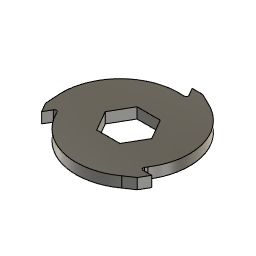
broyeuse V3 v5 (Autodesk Fusion 360 archive; units mm, degrees)
design "Dent A"
Autodesk Fusion 360 part; units mm, degrees
(part 1 of 5)
sketch "Sketch1" plane through (0, 0, 0) normal (0, 0, 1) x (1, 0, 0)
  circle A0 centre (0, 0) radius 25
  dimension "d4" = 50
  constraint coincident A0.centre origin
  measures "d4" diameter of A0
extrude "Extrude1" add sketch "Sketch1" along normal blind 5
sketch "Sketch2" plane through (0, 0, 5) normal (0, 0, 1) x (-1, 0, 0)
  circle A0 centre (0, 0) radius 25
  line L0 (5.4848, -9.5) -> (10.9697, 0)
  line L1 (10.9697, 0) -> (5.4848, 9.5)
  line L2 (5.4848, 9.5) -> (-5.4848, 9.5)
  line L3 (-5.4848, 9.5) -> (-10.9697, 0)
  line L4 (-10.9697, 0) -> (-5.4848, -9.5)
  line L5 (-5.4848, -9.5) -> (5.4848, -9.5)
  dimension "d7" = 19
  constraint coincident A0.centre origin
  measures "d7" distance of L0 L3
extrude "Extrude2" cut sketch "Sketch2" against normal through all contours L0 L1 L2 L3 L4 L5
sketch "Sketch3" plane through (0, 0, 5) normal (0, 0, 1) x (-1, 0, 0)
  line L0 (-10.9697, 0) -> (-5.4848, 9.5)
  line L1 (-5.4848, 9.5) -> (5.4848, 9.5)
  line L2 (5.4848, 9.5) -> (10.9697, 0)
  line L3 (10.9697, 0) -> (5.4848, -9.5)
  line L4 (5.4848, -9.5) -> (-5.4848, -9.5)
  line L5 (-5.4848, -9.5) -> (-10.9697, 0)
  circle A0 centre (0, 0) radius 25
  line L6 (0, -9.5) -> (0, -34) construction
  line L7 (0, -30) -> (-3.0461, -24.8137)
  line L8 (0, 0) -> (-21.6506, 12.5) construction
  arc A1 (-21.6506, 12.5) -> (0, -30) centre (1.3758, -2.5344) ccw
  line L9 (0, -30) -> (-5, -30)
  line L10 (-5, -30) -> (-11.5934, -26.7842)
  dimension "d9" = 120
  dimension "d10" = 55
  dimension "d11" = 30
  dimension "d14" = 5
  dimension "d16" = 154
  constraint midpoint L4 L6.start
  constraint perpendicular L4 L6
  constraint coincident L6 L7.start
  constraint coincident A0 L7.end
  constraint coincident A0.centre L8.start
  constraint coincident A0 L8.end
  constraint perpendicular L6 L9
  constraint coincident A1 L10.end
  measures "d9" angle of L6 L8
  measures "d10" diameter of A1
  measures "d11" distance of L7.start A0.centre
  measures "d14" distance of L7.start L9.end
  measures "d16" angle of L9 L10
extrude "Extrude3" add sketch "Sketch3" against normal blind 5 contours A0 L7 A1 L10 | A1 L10 | A1 L9 L10
pattern_circular "C-Pattern1" count 3 over 360 about axis through (0, 0, 1.75) along (0, 0, 1) of "Extrude3"
fillet "Fillet1" radius 1 3 edges at (19.9663, -15.0449, 2.5) (3.0461, 24.8137, 2.5) (-23.0124, -9.7689, 2.5)
sketch "Sketch4" plane through (0, 0, 5) normal (0, 0, 1) x (-1, 0, 0)
  line L0 (-10.9697, 0) -> (-5.4848, 9.5)
  line L1 (-5.4848, 9.5) -> (5.4848, 9.5)
  line L2 (5.4848, 9.5) -> (10.9697, 0)
  line L3 (10.9697, 0) -> (5.4848, -9.5)
  line L4 (5.4848, -9.5) -> (-5.4848, -9.5)
  line L5 (-5.4848, -9.5) -> (-10.9697, 0)
  arc A0 (-1.1597, -24.9731) -> (0, -25) centre (0, 0) ccw
  arc A1 (0, -25) -> (28.8493, 5.3994) centre (1.507, 2.4587) ccw
  line L6 (28.8493, 5.3994) -> (28.4808, 10.6699)
  line L7 (28.4808, 10.6699) -> (25.9808, 15)
  line L8 (25.9808, 15) -> (23.9652, 11.448)
  arc A2 (22.2072, 11.4822) -> (23.9652, 11.448) centre (23.0955, 11.9415) ccw
  arc A3 (22.2072, 11.4822) -> (21.6506, 12.5) centre (0, 0) ccw
  arc A4 (21.6506, 12.5) -> (-19.1007, 22.2845) centre (-2.8828, 0.0758) ccw
  line L9 (-19.1007, 22.2845) -> (-23.4808, 19.3301)
  line L10 (-23.4808, 19.3301) -> (-25.9808, 15)
  line L11 (-25.9808, 15) -> (-21.8968, 15.0305)
  arc A5 (-21.0475, 13.4909) -> (-21.8968, 15.0305) centre (-21.8894, 14.0305) ccw
  arc A6 (-21.0475, 13.4909) -> (-21.6506, 12.5) centre (0, 0) ccw
  arc A7 (-21.6506, 12.5) -> (-9.7486, -27.6839) centre (1.3758, -2.5344) ccw
  line L12 (-9.7486, -27.6839) -> (-5, -30)
  line L13 (-5, -30) -> (0, -30)
  line L14 (0, -30) -> (-2.0683, -26.4785)
  arc A8 (-1.1597, -24.9731) -> (-2.0683, -26.4785) centre (-1.2061, -25.972) ccw
  line L15 (0, 38) -> (0, -40)
  constraint vertical L15
equation "hexa_dent = 19 mm"
equation "hexa_axe = 19 mm"
equation "d7 = hexa_dent"

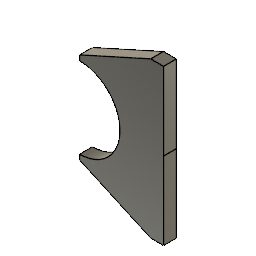
design "entretoise B"
Autodesk Fusion 360 part; units mm, degrees
sketch "Sketch1" plane through (0, 0, 0) normal (0, 1, 0) x (1, 0, 0)
  circle A0 centre (0, 0) radius 14.5 construction
  line L0 (0, -15.6) -> (0, -17.6)
  arc A1 (0, -15.6) -> (15.6, 0) centre (0, 0) ccw
  line L1 (0, -17.6) -> (27.5, -30)
  line L2 (0, 0) -> (15.6, 0) construction
  line L3 (27.5, -30) -> (32.5, -30)
  line L4 (32.5, -30) -> (32.5, 0)
  line L5 (0, -15.6) -> (0, 0) construction
  line L6 (0, 15.6) -> (0, 17.6)
  arc A2 (15.6, 0) -> (0, 15.6) centre (0, 0) ccw
  line L7 (0, 17.6) -> (27.5, 30)
  line L8 (27.5, 30) -> (32.5, 30)
  line L9 (32.5, 30) -> (32.5, 0)
  dimension "d1" = 29
  dimension "d2" = 2
  dimension "d3" = 30
  dimension "d4" = 32.5
  dimension "d5" = 15.6
  dimension "d6" = 5
  constraint coincident A0.centre A1.centre
  constraint horizontal L2
  constraint horizontal L3
  constraint perpendicular L3 L4
  constraint vertical L0
  constraint parallel L0 L5
  constraint symmetric L0.end L2 L6.end
  constraint symmetric L0.start L2 L6.start
  constraint symmetric A1 L2 A2
  constraint symmetric L1.end L2 L7.end
  constraint symmetric L2 A1.end A2.start
  constraint symmetric L2 L3.end L8.end
  constraint symmetric L2 L4.end L9.end
  measures "d1" diameter of A0
  measures "d2" distance of L0.end L0.start
  measures "d3" distance of L2 L3
  measures "d4" distance of A0.centre L4
  measures "d5" radius of A1
  measures "d6" distance of L1.end L3.end
extrude "Extrude1" add sketch "Sketch1" along normal blind 5

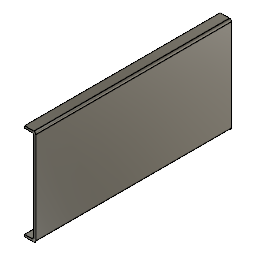
design "Flan"
Autodesk Fusion 360 part; units mm, degrees
sketch "Sketch1" plane through (0, 0, 0) normal (0, 1, 0) x (1, 0, 0)
  line L0 (-8.6431, -45) -> (0.9933, -45)
  line L1 (0.9933, -45) -> (0.9933, 49)
  line L2 (0.9933, 49) -> (-8.6431, 49)
  line L3 (-8.6431, -47.1) -> (3.0933, -47.1)
  line L4 (3.0933, -47.1) -> (3.0933, 51.1)
  line L5 (3.0933, 51.1) -> (-8.6431, 51.1)
  line L6 (-8.6431, -45) -> (-8.6431, -47.1)
  line L7 (-8.6431, 51.1) -> (-8.6431, 49)
  dimension "d1" = 94
  dimension "d2" = 2.1
  constraint horizontal L0
  constraint perpendicular L1 L2
  constraint vertical L1
  constraint equal L0 L2
  constraint perpendicular L2 L7
  measures "d1" distance of L0.end L1.end
extrude "Extrude1" add sketch "Sketch1" along normal blind 200
fillet "Fillet1" radius 2 1 edges at (3.0933, 100, 47.1)
fillet "Fillet1" radius 2 3 edges at (3.0933, 100, -51.1) (0.9933, 100, -49) (0.9933, 100, 45)

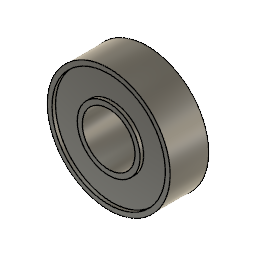
design "Q6202"
Autodesk Fusion 360 part; units mm, degrees
sketch "Sketch1" plane through (0, 0, 0) normal (0, 1, 0) x (1, 0, 0)
  circle A0 centre (0, 0) radius 17.5
  circle A1 centre (0, 0) radius 7.5
  dimension "d1" = 15
  dimension "d2" = 35
  constraint coincident A0.centre A1.centre
  constraint concentric A0 A1
  measures "d1" diameter of A1
  measures "d2" diameter of A0
extrude "Extrude1" add sketch "Sketch1" along normal blind 11
sketch "Sketch2" plane through (0, 0, 0) normal (0, -1, 0) x (1, 0, 0)
  circle A0 centre (0, 0) radius 7.5
  circle A1 centre (0, 0) radius 17.5
  circle A2 centre (0, 0) radius 8.9443
  circle A3 centre (0, 0) radius 16.1245
  constraint concentric A0 A2
  constraint concentric A2 A3
extrude "Extrude2" cut sketch "Sketch2" against normal blind 1 contours A3
ref_plane "WorkPlane1" through (0, 5.5, 0) normal (0, -1, 0) x (-1, 0, 0)
mirror "Mirror1" about plane through (0, 5.5, 0) normal (0, -1, 0) of "Extrude2"

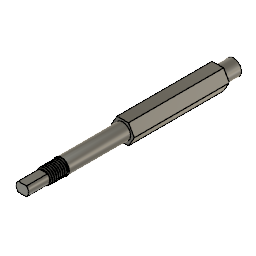
design "axe B"
Autodesk Fusion 360 part; units mm, degrees
sketch "Sketch1" plane through (0, 0, 0) normal (0, 1, 0) x (1, 0, 0)
  line L0 (5.4848, -9.5) -> (10.9697, 0)
  line L1 (10.9697, 0) -> (5.4848, 9.5)
  line L2 (5.4848, 9.5) -> (-5.4848, 9.5)
  line L3 (-5.4848, 9.5) -> (-10.9697, 0)
  line L4 (-10.9697, 0) -> (-5.4848, -9.5)
  line L5 (-5.4848, -9.5) -> (5.4848, -9.5)
  dimension "d1" = 19
  measures "d1" distance of L1 L4
extrude "Extrude1" add sketch "Sketch1" along normal blind 90
sketch "Sketch2" plane through (0, 0, 0) normal (0, -1, 0) x (1, 0, 0)
  line L0 (5.4848, 9.5) -> (-5.4848, 9.5)
  line L1 (-5.4848, 9.5) -> (-10.9697, 0)
  line L2 (-10.9697, 0) -> (-5.4848, -9.5)
  line L3 (-5.4848, -9.5) -> (5.4848, -9.5)
  line L4 (5.4848, -9.5) -> (10.9697, 0)
  line L5 (10.9697, 0) -> (5.4848, 9.5)
  circle A0 centre (0, 0) radius 7.5
  dimension "d4" = 15
  constraint coincident A0.centre origin
  measures "d4" diameter of A0
extrude "Extrude2" add sketch "Sketch2" along normal blind 58 contours A0
sketch "Sketch3" plane through (0, -58, 0) normal (0, -1, 0) x (1, 0, 0)
  circle A0 centre (0, 0) radius 7.5
  circle A1 centre (0, 0) radius 7
  dimension "d7" = 14
  constraint concentric A0 A1
  measures "d7" diameter of A1
extrude "Extrude3" add sketch "Sketch3" along normal blind 17 contours A1
thread "Thread1" "ISO Metric profile 14.0 M14x2 6g" major diameter 13.822 minor diameter 11.534 pitch 2 angle 60 modelled right hand crest width 0.2847 on face at (6.9913, -69.3333, -0.3489) crest through (6.911, -57.5, 0)
sketch "Sketch4" plane through (0, 90, 0) normal (0, 1, 0) x (-1, 0, 0)
  line L0 (5.4848, 9.5) -> (-5.4848, 9.5)
  line L1 (-5.4848, 9.5) -> (-10.9697, 0)
  line L2 (-10.9697, 0) -> (-5.4848, -9.5)
  line L3 (-5.4848, -9.5) -> (5.4848, -9.5)
  line L4 (5.4848, -9.5) -> (10.9697, 0)
  line L5 (10.9697, 0) -> (5.4848, 9.5)
  circle A0 centre (0, 0) radius 7.5
  dimension "d10" = 15
  constraint coincident A0.centre origin
  measures "d10" diameter of A0
extrude "Extrude4" add sketch "Sketch4" along normal blind 15 contours A0
sketch "Sketch5" plane through (0, -75, 0) normal (0, -1, 0) x (1, 0, 0)
  spline S0 degree 3 poles (-3.3483, 4.6955) (-4.0071, 4.3146) (-4.5838, 3.8067) (-5.5311, 2.5793) (-5.8844, 1.8654) (-6.3098, 0.3166) (-6.3676, -0.506) (-6.1666, -2.1557) (-5.8992, -2.9654) (-5.1959, -4.2209) (-4.8371, -4.6975) (-3.9949, -5.5534) (-3.5129, -5.9264) (-2.9883, -6.2315) knots 0 0 0 0 0.228303 0.228303 0.464774 0.464774 0.709409 0.709409 0.962206 0.962206 1.139841 1.139841 1.321288 1.321288 1.321288 1.321288
  arc A0 (-2.9883, -6.2315) -> (2.9883, -6.2315) centre (0, 0) ccw
  spline S1 degree 3 poles (2.9883, -6.2315) (3.7522, -5.7873) (4.4234, -5.2003) (5.482, -3.8207) (5.8675, -3.048) (6.3085, -1.4236) (6.3697, -0.5904) (6.1676, 1.0246) (5.9167, 1.7919) (5.2631, 2.9496) (4.9429, 3.3747) (4.2065, 4.1187) (3.7959, 4.4367) (3.3483, 4.6955) knots 0 0 0 0 0.265106 0.265106 0.522028 0.522028 0.770763 0.770763 1.011307 1.011307 1.170725 1.170725 1.326339 1.326339 1.326339 1.326339
  arc A1 (3.3483, 4.6955) -> (-3.3483, 4.6955) centre (0, 0) ccw
  circle A2 centre (0, 0) radius 6
  dimension "d13" = 12
  constraint coincident A0.centre A1.centre
  measures "d13" diameter of A2
extrude "Extrude5" add sketch "Sketch5" along normal blind 20 contours S0 S1 A1 A2 | S0 S1 A1 A2
sketch "Sketch6" plane through (0, -95, 0) normal (0, -1, 0) x (1, 0, 0)
  circle A0 centre (0, 0) radius 6
  line L0 (0, 0) -> (0, 6) construction
  line L1 (-8, 9.5) -> (10.7231, 9.5)
  line L2 (10.7231, 9.5) -> (10.7231, 4.5)
  line L3 (10.7231, 4.5) -> (-8, 4.5)
  line L4 (-8, 4.5) -> (-8, 9.5)
  line L5 (0, 0) -> (17.434, 0) construction
  line L6 (10.7231, -4.5) -> (-8, -4.5)
  line L7 (-8, -4.5) -> (-8, -9.5)
  line L8 (-8, -9.5) -> (10.7231, -9.5)
  line L9 (10.7231, -9.5) -> (10.7231, -4.5)
  dimension "d16" = 5
  dimension "d17" = 1.5
  constraint coincident A0.centre L0.start
  constraint vertical L0
  constraint horizontal L1
  constraint vertical L2
  constraint horizontal L3
  constraint vertical L4
  constraint coincident A0 L0.end
  constraint perpendicular L0 L5
  constraint symmetric L1.start L5 L7.end
  constraint symmetric L1.end L5 L8.end
  constraint symmetric L2.end L5 L6.start
  constraint symmetric L3.end L5 L6.end
  measures "d16" distance of L1.end L2.end
  measures "d17" distance of L0.end L3
extrude "Extrude6" cut sketch "Sketch6" against normal blind 20 contours A0 L3 | A0 L6

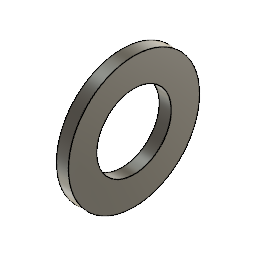
design "rondelle étroite M14 forme Z"
Autodesk Fusion 360 part; units mm, degrees
sketch "Sketch1" plane through (0, 0, 0) normal (1, 0, 0) x (0, 1, 0)
  circle A0 centre (0, 0) radius 7.65
  circle A1 centre (0, 0) radius 13.5
  dimension "d1" = 15.3
  dimension "d2" = 27
  constraint coincident A0.centre A1.centre
  measures "d1" diameter of A0
  measures "d2" diameter of A1
extrude "Extrude1" add sketch "Sketch1" along normal blind 2.5

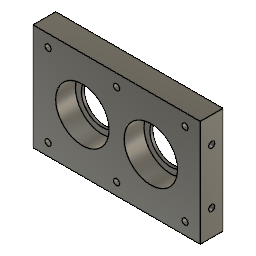
design "Plaque facade A"
Autodesk Fusion 360 part; units mm, degrees
sketch "Sketch1" plane through (0, 0, 0) normal (0, 1, 0) x (1, 0, 0)
  circle A0 centre (-22.5, 0) radius 13.6
  circle A1 centre (22.5, 0) radius 13.6
  line L0 (-22.5, 0) -> (22.5, 0) construction
  line L1 (0, 0) -> (0, -35) construction
  line L2 (-55, -35) -> (55, -35)
  line L3 (55, -35) -> (55, 35)
  line L4 (55, 35) -> (-55, 35)
  line L5 (-55, 35) -> (-55, -35)
  line L6 (-55, 0) -> (-22.5, 0) construction
  dimension "d1" = 27.2
  dimension "d2" = 45
  dimension "d3" = 70
  dimension "d4" = 110
  constraint equal A0 A1
  constraint coincident A0.centre L0.start
  constraint coincident A1.centre L0.end
  constraint horizontal L0
  constraint midpoint L0 L1.start
  constraint perpendicular L0 L1
  constraint coincident L1.start origin
  constraint horizontal L2
  constraint vertical L3
  constraint horizontal L4
  constraint vertical L5
  constraint midpoint L5 L6.start
  constraint perpendicular L5 L6
  constraint midpoint L1.end L2
  measures "d1" diameter of A0
  measures "d2" distance of A0.centre A1.centre
  measures "d3" distance of L2.start L4.end
  measures "d4" distance of L2.start L2.end
extrude "Extrude1" add sketch "Sketch1" along normal blind 15
sketch "Sketch2" plane through (0, 0, 0) normal (0, -1, 0) x (1, 0, 0)
  circle A0 centre (-22.5, 0) radius 13.6
  circle A1 centre (22.5, 0) radius 13.6
  line L0 (-55, 35) -> (-55, -35)
  line L1 (-55, -35) -> (55, -35)
  line L2 (55, -35) -> (55, 35)
  line L3 (55, 35) -> (-55, 35)
  circle A2 centre (-22.5, 0) radius 17.5
  circle A3 centre (22.5, 0) radius 17.5
  dimension "d7" = 35
  constraint concentric A0 A2
  constraint concentric A1 A3
  constraint equal A2 A3
  measures "d7" diameter of A2
extrude "Extrude2" cut sketch "Sketch2" against normal blind 13 contours A2 | A3
sketch "Sketch3" plane through (55, 0, 0) normal (1, 0, 0) x (0, 1, 0)
  line L0 (0, 35) -> (0, -35)
  line L1 (0, -35) -> (15, -35)
  line L2 (15, -35) -> (15, 35)
  line L3 (15, 35) -> (0, 35)
  line L4 (7.5, 35) -> (7.5, -35) construction
  circle A0 centre (7.5, 18) radius 2
  circle A1 centre (7.5, -18) radius 2
  line L5 (7.5, 0) -> (33, 0) construction
  dimension "d10" = 4
  dimension "d11" = 18
  dimension "d12" = 18
  constraint midpoint L3 L4.start
  constraint midpoint L1 L4.end
  constraint coincident L4 A0.centre
  constraint coincident L4 A1.centre
  constraint equal A0 A1
  constraint midpoint L4 L5.start
  constraint perpendicular L2 L5
  measures "d10" diameter of A0
  measures "d11" distance of A0.centre L5
  measures "d12" distance of A1.centre L5.start
extrude "Extrude3" cut sketch "Sketch3" against normal blind 20 contours A0 | A1
ref_plane "WorkPlane1" through (0, 7.5, 0) normal (1, 0, 0) x (0, 0, -1)
mirror "Mirror1" about plane through (0, 7.5, 0) normal (1, 0, 0) of "Extrude3"
sketch "Sketch4" plane through (0, 0, 0) normal (0, -1, 0) x (1, 0, 0)
  circle A0 centre (-22.5, 0) radius 17.5
  circle A1 centre (22.5, 0) radius 17.5
  line L0 (-55, 35) -> (-55, -35)
  line L1 (-55, -35) -> (55, -35)
  line L2 (55, -35) -> (55, 35)
  line L3 (55, 35) -> (-55, 35)
  line L4 (-55, 27) -> (55, 27) construction
  circle A2 centre (0, 27) radius 2
  circle A3 centre (-45, 27) radius 2
  circle A4 centre (45, 27) radius 2
  line L5 (55, 0) -> (-55, 0) construction
  circle A5 centre (45, -27) radius 2
  circle A6 centre (0, -27) radius 2
  circle A7 centre (-45, -27) radius 2
  dimension "d16" = 4
  dimension "d17" = 10
  dimension "d18" = 10
  dimension "d20" = 8
  constraint coincident L0 L4.start
  constraint coincident L2 L4.end
  constraint perpendicular L2 L4
  constraint midpoint L4 A2.centre
  constraint coincident L4 A3.centre
  constraint coincident L4 A4.centre
  constraint equal A2 A4
  constraint equal A2 A3
  constraint midpoint L2 L5.start
  constraint midpoint L0 L5.end
  constraint symmetric A2 L5 A6
  constraint symmetric A3 L5 A7
  constraint symmetric A4 L5 A5
  measures "d16" diameter of A3
  measures "d17" distance of L0 A3.centre
  measures "d18" distance of L2 A4.centre
  measures "d20" distance of L3 L4
extrude "Extrude4" cut sketch "Sketch4" against normal through all contours A2 | A3 | A4 | A5 | A6 | A7
equation "d12 = d11"

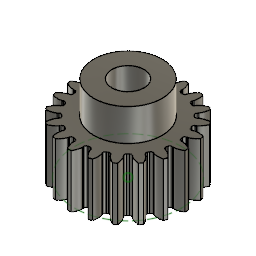
design "Engrenage 16D M2,5"
description: Spur Gear; Module: 2.5; Num Teeth: 20; Pressure Angle: 20.0; Backlash: 0.00 mm
Autodesk Fusion 360 part; units mm, degrees
sketch "Sketch1" plane through (0, 0, 0) normal (0, 0, 1) x (1, 0, 0) in component "Spur Gear (20 teeth)"
  circle A0 centre (0, 0) radius 21.9492
  circle A1 centre (0, 0) radius 7.5
extrude "Extrude1" add sketch "Sketch1" along normal blind 25 in component "Spur Gear (20 teeth)"
sketch "Sketch2" plane through (0, 0, 0) normal (0, 0, 1) x (1, 0, 0) in component "Spur Gear (20 teeth)"
  spline S0 degree 5 poles (23.3898, -2.192) (23.4016, -2.1931) (23.4251, -2.195) (23.4604, -2.1969) (23.5076, -2.1976) (23.5666, -2.1961) (23.6257, -2.1928) (23.6849, -2.1885) (23.7441, -2.1835) (23.8033, -2.1781) (23.8626, -2.1724) (23.9218, -2.166) (23.9811, -2.159) (24.0404, -2.151) (24.0996, -2.1423) (24.1589, -2.1327) (24.2182, -2.1224) (24.2775, -2.1116) (24.3368, -2.1003) (24.396, -2.0885) (24.4553, -2.0763) (24.5145, -2.0635) (24.5737, -2.0503) (24.6329, -2.0365) (24.6921, -2.0221) (24.7513, -2.0073) (24.8104, -1.992) (24.8696, -1.9762) (24.9287, -1.96) (24.9877, -1.9433) (25.0468, -1.9262) (25.1058, -1.9087) (25.1648, -1.8908) (25.2237, -1.8724) (25.2826, -1.8536) (25.3415, -1.8344) (25.4004, -1.8148) (25.4592, -1.7947) (25.518, -1.7743) (25.5767, -1.7535) (25.6354, -1.7323) (25.694, -1.7108) (25.7526, -1.6888) (25.8112, -1.6665) (25.8697, -1.6438) (25.9282, -1.6207) (25.9866, -1.5972) (26.045, -1.5734) (26.1034, -1.5493) (26.1616, -1.5248) (26.2199, -1.4999) (26.2781, -1.4747) (26.3362, -1.4491) (26.3943, -1.4232) (26.4523, -1.3969) (26.5102, -1.3704) (26.5682, -1.3434) (26.626, -1.3162) (26.6838, -1.2886) (26.7415, -1.2606) (26.7992, -1.2324) (26.8568, -1.2038) (26.9144, -1.1749) (26.9719, -1.1457) (27.0293, -1.1161) (27.0866, -1.0863) (27.1439, -1.0561) (27.2012, -1.0256) (27.2583, -0.9948) (27.3154, -0.9637) (27.3725, -0.9323) (27.418, -0.9069) (27.4522, -0.8877) (27.4749, -0.8749) (27.4863, -0.8685) knots 0 0 0 0 0 0 0.01428571 0.02857143 0.04285714 0.05714286 0.07142857 0.08571429 0.1 0.11428571 0.12857143 0.14285714 0.15714286 0.17142857 0.18571429 0.2 0.21428571 0.22857143 0.24285714 0.25714286 0.27142857 0.28571429 0.3 0.31428571 0.32857143 0.34285714 0.35714286 0.37142857 0.38571429 0.4 0.41428571 0.42857143 0.44285714 0.45714286 0.47142857 0.48571429 0.5 0.51428571 0.52857143 0.54285714 0.55714286 0.57142857 0.58571429 0.6 0.61428571 0.62857143 0.64285714 0.65714286 0.67142857 0.68571429 0.7 0.71428571 0.72857143 0.74285714 0.75714286 0.77142857 0.78571429 0.8 0.81428571 0.82857143 0.84285714 0.85714286 0.87142857 0.88571429 0.9 0.91428571 0.92857143 0.94285714 0.95714286 0.97142857 0.98571429 1 1 1 1 1 1
  spline S1 degree 5 poles (23.3898, 2.192) (23.4016, 2.1931) (23.4251, 2.195) (23.4604, 2.1969) (23.5076, 2.1976) (23.5666, 2.1961) (23.6257, 2.1928) (23.6849, 2.1885) (23.7441, 2.1835) (23.8033, 2.1781) (23.8626, 2.1724) (23.9218, 2.166) (23.9811, 2.159) (24.0404, 2.151) (24.0996, 2.1423) (24.1589, 2.1327) (24.2182, 2.1224) (24.2775, 2.1116) (24.3368, 2.1003) (24.396, 2.0885) (24.4553, 2.0763) (24.5145, 2.0635) (24.5737, 2.0503) (24.6329, 2.0365) (24.6921, 2.0221) (24.7513, 2.0073) (24.8104, 1.992) (24.8696, 1.9762) (24.9287, 1.96) (24.9877, 1.9433) (25.0468, 1.9262) (25.1058, 1.9087) (25.1648, 1.8908) (25.2237, 1.8724) (25.2826, 1.8536) (25.3415, 1.8344) (25.4004, 1.8148) (25.4592, 1.7947) (25.518, 1.7743) (25.5767, 1.7535) (25.6354, 1.7323) (25.694, 1.7108) (25.7526, 1.6888) (25.8112, 1.6665) (25.8697, 1.6438) (25.9282, 1.6207) (25.9866, 1.5972) (26.045, 1.5734) (26.1034, 1.5493) (26.1616, 1.5248) (26.2199, 1.4999) (26.2781, 1.4747) (26.3362, 1.4491) (26.3943, 1.4232) (26.4523, 1.3969) (26.5102, 1.3704) (26.5682, 1.3434) (26.626, 1.3162) (26.6838, 1.2886) (26.7415, 1.2606) (26.7992, 1.2324) (26.8568, 1.2038) (26.9144, 1.1749) (26.9719, 1.1457) (27.0293, 1.1161) (27.0866, 1.0863) (27.1439, 1.0561) (27.2012, 1.0256) (27.2583, 0.9948) (27.3154, 0.9637) (27.3725, 0.9323) (27.418, 0.9069) (27.4522, 0.8877) (27.4749, 0.8749) (27.4863, 0.8685) knots 0 0 0 0 0 0 0.01428571 0.02857143 0.04285714 0.05714286 0.07142857 0.08571429 0.1 0.11428571 0.12857143 0.14285714 0.15714286 0.17142857 0.18571429 0.2 0.21428571 0.22857143 0.24285714 0.25714286 0.27142857 0.28571429 0.3 0.31428571 0.32857143 0.34285714 0.35714286 0.37142857 0.38571429 0.4 0.41428571 0.42857143 0.44285714 0.45714286 0.47142857 0.48571429 0.5 0.51428571 0.52857143 0.54285714 0.55714286 0.57142857 0.58571429 0.6 0.61428571 0.62857143 0.64285714 0.65714286 0.67142857 0.68571429 0.7 0.71428571 0.72857143 0.74285714 0.75714286 0.77142857 0.78571429 0.8 0.81428571 0.82857143 0.84285714 0.85714286 0.87142857 0.88571429 0.9 0.91428571 0.92857143 0.94285714 0.95714286 0.97142857 0.98571429 1 1 1 1 1 1
  arc A0 (27.4863, -0.8685) -> (27.4863, 0.8685) centre (0, 0) ccw
  line L0 (21.8435, -2.048) -> (23.3898, -2.192)
  line L1 (21.8435, 2.048) -> (23.3898, 2.192)
  line L2 (21.8435, -2.048) -> (21.8435, 2.048)
  point P0 (23.6776, -2.1889)
  point P1 (23.9677, -2.1604)
  point P2 (24.2591, -2.1149)
  point P3 (24.5515, -2.0552)
  point P4 (24.8446, -1.9828)
  point P5 (25.1383, -1.8988)
  point P6 (25.4323, -1.8039)
  point P7 (25.7264, -1.6986)
  point P8 (26.0206, -1.5834)
  point P9 (26.3146, -1.4586)
  point P10 (26.6083, -1.3245)
  point P11 (26.9016, -1.1813)
  point P12 (27.1943, -1.0292)
  point P13 (23.6776, 2.1889)
  point P14 (23.9677, 2.1604)
  point P15 (24.2591, 2.1149)
  point P16 (24.5515, 2.0552)
  point P17 (24.8446, 1.9828)
  point P18 (25.1383, 1.8988)
  point P19 (25.4323, 1.8039)
  point P20 (25.7264, 1.6986)
  point P21 (26.0206, 1.5834)
  point P22 (26.3146, 1.4586)
  point P23 (26.6083, 1.3245)
  point P24 (26.9016, 1.1813)
  point P25 (27.1943, 1.0292)
extrude "Extrude2" add sketch "Sketch2" along normal blind 25 in component "Spur Gear (20 teeth)"
fillet "Fillet1" radius 1 2 edges at (21.8534, -2.049, 12.5) (21.8534, 2.049, 12.5) in component "Spur Gear (20 teeth)"
pattern_circular "C-Pattern1" count 20 over 360 about axis through (0, 0, 0) along (0, 0, 1) of "Extrude2", "Fillet1" in component "Spur Gear (20 teeth)"
sketch "Sketch3" plane through (0, 0, 0) normal (0, 0, 1) x (1, 0, 0) in component "Spur Gear (20 teeth)"
  circle A0 centre (0, 0) radius 25 construction
sketch "Sketch1 (2)" plane through (0, 0, 25) normal (0, 0, 1) x (-1, 0, 0)
  arc A0 (-21.6058, 3.8672) -> (-21.7434, 2.9987) centre (0, 0) ccw
  arc A1 (-22.8267, 2.1396) -> (-21.7434, 2.9987) centre (-22.734, 3.1353) ccw
  line L0 (-22.8267, 2.1396) -> (-23.3898, 2.192)
  spline S0 degree 5 poles (-23.3898, 2.192) (-23.4016, 2.1931) (-23.4251, 2.195) (-23.4604, 2.1969) (-23.5076, 2.1976) (-23.5666, 2.1961) (-23.6257, 2.1928) (-23.6849, 2.1885) (-23.7441, 2.1835) (-23.8033, 2.1781) (-23.8626, 2.1724) (-23.9218, 2.166) (-23.9811, 2.159) (-24.0404, 2.151) (-24.0996, 2.1423) (-24.1589, 2.1327) (-24.2182, 2.1224) (-24.2775, 2.1116) (-24.3368, 2.1003) (-24.396, 2.0885) (-24.4553, 2.0763) (-24.5145, 2.0635) (-24.5737, 2.0503) (-24.6329, 2.0365) (-24.6921, 2.0221) (-24.7513, 2.0073) (-24.8104, 1.992) (-24.8696, 1.9762) (-24.9287, 1.96) (-24.9877, 1.9433) (-25.0468, 1.9262) (-25.1058, 1.9087) (-25.1648, 1.8908) (-25.2237, 1.8724) (-25.2826, 1.8536) (-25.3415, 1.8344) (-25.4004, 1.8148) (-25.4592, 1.7947) (-25.518, 1.7743) (-25.5767, 1.7535) (-25.6354, 1.7323) (-25.694, 1.7108) (-25.7526, 1.6888) (-25.8112, 1.6665) (-25.8697, 1.6438) (-25.9282, 1.6207) (-25.9866, 1.5972) (-26.045, 1.5734) (-26.1034, 1.5493) (-26.1616, 1.5248) (-26.2199, 1.4999) (-26.2781, 1.4747) (-26.3362, 1.4491) (-26.3943, 1.4232) (-26.4523, 1.3969) (-26.5102, 1.3704) (-26.5682, 1.3434) (-26.626, 1.3162) (-26.6838, 1.2886) (-26.7415, 1.2606) (-26.7992, 1.2324) (-26.8568, 1.2038) (-26.9144, 1.1749) (-26.9719, 1.1457) (-27.0293, 1.1161) (-27.0866, 1.0863) (-27.1439, 1.0561) (-27.2012, 1.0256) (-27.2583, 0.9948) (-27.3154, 0.9637) (-27.3725, 0.9323) (-27.418, 0.9069) (-27.4522, 0.8877) (-27.4749, 0.8749) (-27.4863, 0.8685) knots 0 0 0 0 0 0 0.01428571 0.02857143 0.04285714 0.05714286 0.07142857 0.08571429 0.1 0.11428571 0.12857143 0.14285714 0.15714286 0.17142857 0.18571429 0.2 0.21428571 0.22857143 0.24285714 0.25714286 0.27142857 0.28571429 0.3 0.31428571 0.32857143 0.34285714 0.35714286 0.37142857 0.38571429 0.4 0.41428571 0.42857143 0.44285714 0.45714286 0.47142857 0.48571429 0.5 0.51428571 0.52857143 0.54285714 0.55714286 0.57142857 0.58571429 0.6 0.61428571 0.62857143 0.64285714 0.65714286 0.67142857 0.68571429 0.7 0.71428571 0.72857143 0.74285714 0.75714286 0.77142857 0.78571429 0.8 0.81428571 0.82857143 0.84285714 0.85714286 0.87142857 0.88571429 0.9 0.91428571 0.92857143 0.94285714 0.95714286 0.97142857 0.98571429 1 1 1 1 1 1
  arc A2 (-27.4863, 0.8685) -> (-27.4863, -0.8685) centre (0, 0) ccw
  spline S1 degree 5 poles (-27.4863, -0.8685) (-27.4749, -0.8749) (-27.4522, -0.8877) (-27.418, -0.9069) (-27.3725, -0.9323) (-27.3154, -0.9637) (-27.2583, -0.9948) (-27.2012, -1.0256) (-27.1439, -1.0561) (-27.0866, -1.0863) (-27.0293, -1.1161) (-26.9719, -1.1457) (-26.9144, -1.1749) (-26.8568, -1.2038) (-26.7992, -1.2324) (-26.7415, -1.2606) (-26.6838, -1.2886) (-26.626, -1.3162) (-26.5682, -1.3434) (-26.5102, -1.3704) (-26.4523, -1.3969) (-26.3943, -1.4232) (-26.3362, -1.4491) (-26.2781, -1.4747) (-26.2199, -1.4999) (-26.1616, -1.5248) (-26.1034, -1.5493) (-26.045, -1.5734) (-25.9866, -1.5972) (-25.9282, -1.6207) (-25.8697, -1.6438) (-25.8112, -1.6665) (-25.7526, -1.6888) (-25.694, -1.7108) (-25.6354, -1.7323) (-25.5767, -1.7535) (-25.518, -1.7743) (-25.4592, -1.7947) (-25.4004, -1.8148) (-25.3415, -1.8344) (-25.2826, -1.8536) (-25.2237, -1.8724) (-25.1648, -1.8908) (-25.1058, -1.9087) (-25.0468, -1.9262) (-24.9877, -1.9433) (-24.9287, -1.96) (-24.8696, -1.9762) (-24.8104, -1.992) (-24.7513, -2.0073) (-24.6921, -2.0221) (-24.6329, -2.0365) (-24.5737, -2.0503) (-24.5145, -2.0635) (-24.4553, -2.0763) (-24.396, -2.0885) (-24.3368, -2.1003) (-24.2775, -2.1116) (-24.2182, -2.1224) (-24.1589, -2.1327) (-24.0996, -2.1423) (-24.0404, -2.151) (-23.9811, -2.159) (-23.9218, -2.166) (-23.8626, -2.1724) (-23.8033, -2.1781) (-23.7441, -2.1835) (-23.6849, -2.1885) (-23.6257, -2.1928) (-23.5666, -2.1961) (-23.5076, -2.1976) (-23.4604, -2.1969) (-23.4251, -2.195) (-23.4016, -2.1931) (-23.3898, -2.192) knots -1 -1 -1 -1 -1 -1 -0.98571429 -0.97142857 -0.95714286 -0.94285714 -0.92857143 -0.91428571 -0.9 -0.88571429 -0.87142857 -0.85714286 -0.84285714 -0.82857143 -0.81428571 -0.8 -0.78571429 -0.77142857 -0.75714286 -0.74285714 -0.72857143 -0.71428571 -0.7 -0.68571429 -0.67142857 -0.65714286 -0.64285714 -0.62857143 -0.61428571 -0.6 -0.58571429 -0.57142857 -0.55714286 -0.54285714 -0.52857143 -0.51428571 -0.5 -0.48571429 -0.47142857 -0.45714286 -0.44285714 -0.42857143 -0.41428571 -0.4 -0.38571429 -0.37142857 -0.35714286 -0.34285714 -0.32857143 -0.31428571 -0.3 -0.28571429 -0.27142857 -0.25714286 -0.24285714 -0.22857143 -0.21428571 -0.2 -0.18571429 -0.17142857 -0.15714286 -0.14285714 -0.12857143 -0.11428571 -0.1 -0.08571429 -0.07142857 -0.05714286 -0.04285714 -0.02857143 -0.01428571 0 0 0 0 0 0
  line L1 (-23.3898, -2.192) -> (-22.8267, -2.1396)
  arc A3 (-21.7434, -2.9987) -> (-22.8267, -2.1396) centre (-22.734, -3.1353) ccw
  arc A4 (-21.7434, -2.9987) -> (-21.6058, -3.8672) centre (0, 0) ccw
  arc A5 (-22.3707, -5.019) -> (-21.6058, -3.8672) centre (-22.5902, -4.0434) ccw
  line L2 (-22.3707, -5.019) -> (-22.9224, -5.1431)
  spline S2 degree 5 poles (-22.9224, -5.1431) (-22.9339, -5.1457) (-22.9569, -5.1512) (-22.9911, -5.1603) (-23.0361, -5.1742) (-23.0918, -5.1939) (-23.147, -5.2153) (-23.2019, -5.2377) (-23.2567, -5.2607) (-23.3114, -5.2841) (-23.3659, -5.3079) (-23.4203, -5.3322) (-23.4745, -5.3573) (-23.5284, -5.3831) (-23.5821, -5.4098) (-23.6355, -5.4372) (-23.6888, -5.4653) (-23.7418, -5.4939) (-23.7947, -5.523) (-23.8474, -5.5525) (-23.9, -5.5824) (-23.9523, -5.6129) (-24.0046, -5.6438) (-24.0566, -5.6752) (-24.1085, -5.7071) (-24.1602, -5.7395) (-24.2117, -5.7724) (-24.263, -5.8056) (-24.3142, -5.8393) (-24.3653, -5.8734) (-24.4161, -5.9079) (-24.4668, -5.9428) (-24.5174, -5.9781) (-24.5678, -6.0138) (-24.618, -6.0499) (-24.6681, -6.0864) (-24.718, -6.1232) (-24.7677, -6.1604) (-24.8173, -6.198) (-24.8667, -6.2359) (-24.916, -6.2742) (-24.9651, -6.3129) (-25.0141, -6.3519) (-25.0629, -6.3912) (-25.1115, -6.4309) (-25.16, -6.4709) (-25.2083, -6.5112) (-25.2565, -6.5519) (-25.3045, -6.5929) (-25.3524, -6.6343) (-25.4001, -6.6759) (-25.4476, -6.7179) (-25.495, -6.7601) (-25.5422, -6.8027) (-25.5893, -6.8456) (-25.6362, -6.8888) (-25.683, -6.9323) (-25.7296, -6.9761) (-25.776, -7.0202) (-25.8223, -7.0646) (-25.8684, -7.1093) (-25.9144, -7.1543) (-25.9602, -7.1996) (-26.0058, -7.2452) (-26.0513, -7.291) (-26.0966, -7.3371) (-26.1418, -7.3835) (-26.1868, -7.4302) (-26.2316, -7.4772) (-26.2763, -7.5244) (-26.3208, -7.5719) (-26.3563, -7.6101) (-26.3829, -7.6389) (-26.4006, -7.6581) (-26.4094, -7.6678) knots 0 0 0 0 0 0 0.01428571 0.02857143 0.04285714 0.05714286 0.07142857 0.08571429 0.1 0.11428571 0.12857143 0.14285714 0.15714286 0.17142857 0.18571429 0.2 0.21428571 0.22857143 0.24285714 0.25714286 0.27142857 0.28571429 0.3 0.31428571 0.32857143 0.34285714 0.35714286 0.37142857 0.38571429 0.4 0.41428571 0.42857143 0.44285714 0.45714286 0.47142857 0.48571429 0.5 0.51428571 0.52857143 0.54285714 0.55714286 0.57142857 0.58571429 0.6 0.61428571 0.62857143 0.64285714 0.65714286 0.67142857 0.68571429 0.7 0.71428571 0.72857143 0.74285714 0.75714286 0.77142857 0.78571429 0.8 0.81428571 0.82857143 0.84285714 0.85714286 0.87142857 0.88571429 0.9 0.91428571 0.92857143 0.94285714 0.95714286 0.97142857 0.98571429 1 1 1 1 1 1
  arc A6 (-26.4094, -7.6678) -> (-25.8726, -9.3197) centre (0, 0) ccw
  spline S3 degree 5 poles (-25.8726, -9.3197) (-25.8598, -9.3223) (-25.8342, -9.3275) (-25.7958, -9.3352) (-25.7447, -9.3452) (-25.6807, -9.3575) (-25.6168, -9.3694) (-25.5529, -9.381) (-25.4891, -9.3924) (-25.4253, -9.4033) (-25.3615, -9.414) (-25.2977, -9.4244) (-25.234, -9.4344) (-25.1704, -9.4441) (-25.1067, -9.4535) (-25.0432, -9.4625) (-24.9796, -9.4712) (-24.9161, -9.4796) (-24.8527, -9.4877) (-24.7893, -9.4954) (-24.7259, -9.5028) (-24.6626, -9.5098) (-24.5994, -9.5165) (-24.5362, -9.5229) (-24.4731, -9.5289) (-24.41, -9.5345) (-24.347, -9.5398) (-24.2841, -9.5448) (-24.2212, -9.5494) (-24.1584, -9.5536) (-24.0956, -9.5575) (-24.033, -9.561) (-23.9704, -9.5642) (-23.9078, -9.5669) (-23.8454, -9.5693) (-23.783, -9.5713) (-23.7207, -9.573) (-23.6585, -9.5742) (-23.5964, -9.5751) (-23.5344, -9.5756) (-23.4724, -9.5756) (-23.4106, -9.5753) (-23.3488, -9.5746) (-23.2872, -9.5734) (-23.2257, -9.5718) (-23.1642, -9.5698) (-23.1029, -9.5674) (-23.0417, -9.5646) (-22.9806, -9.5613) (-22.9196, -9.5576) (-22.8587, -9.5535) (-22.798, -9.5488) (-22.7374, -9.5436) (-22.677, -9.5379) (-22.6167, -9.5318) (-22.5566, -9.5251) (-22.4966, -9.518) (-22.4367, -9.5104) (-22.377, -9.5024) (-22.3175, -9.4938) (-22.2581, -9.4846) (-22.199, -9.4746) (-22.1402, -9.4638) (-22.0817, -9.4523) (-22.0233, -9.44) (-21.9652, -9.4272) (-21.9072, -9.414) (-21.8494, -9.4004) (-21.7918, -9.3863) (-21.7346, -9.3711) (-21.6779, -9.3543) (-21.6333, -9.339) (-21.6003, -9.3263) (-21.5785, -9.3173) (-21.5677, -9.3126) knots -1 -1 -1 -1 -1 -1 -0.98571429 -0.97142857 -0.95714286 -0.94285714 -0.92857143 -0.91428571 -0.9 -0.88571429 -0.87142857 -0.85714286 -0.84285714 -0.82857143 -0.81428571 -0.8 -0.78571429 -0.77142857 -0.75714286 -0.74285714 -0.72857143 -0.71428571 -0.7 -0.68571429 -0.67142857 -0.65714286 -0.64285714 -0.62857143 -0.61428571 -0.6 -0.58571429 -0.57142857 -0.55714286 -0.54285714 -0.52857143 -0.51428571 -0.5 -0.48571429 -0.47142857 -0.45714286 -0.44285714 -0.42857143 -0.41428571 -0.4 -0.38571429 -0.37142857 -0.35714286 -0.34285714 -0.32857143 -0.31428571 -0.3 -0.28571429 -0.27142857 -0.25714286 -0.24285714 -0.22857143 -0.21428571 -0.2 -0.18571429 -0.17142857 -0.15714286 -0.14285714 -0.12857143 -0.11428571 -0.1 -0.08571429 -0.07142857 -0.05714286 -0.04285714 -0.02857143 -0.01428571 0 0 0 0 0 0
  line L3 (-21.5677, -9.3126) -> (-21.0483, -9.0887)
  arc A7 (-19.7526, -9.571) -> (-21.0483, -9.0887) centre (-20.6525, -10.007) ccw
  arc A8 (-19.7526, -9.571) -> (-19.3534, -10.3545) centre (0, 0) ccw
  arc A9 (-19.7248, -11.6862) -> (-19.3534, -10.3545) centre (-20.2351, -10.8262) ccw
  line L4 (-19.7248, -11.6862) -> (-20.2112, -11.9748)
  spline S4 degree 5 poles (-20.2112, -11.9748) (-20.2214, -11.9808) (-20.2415, -11.9931) (-20.2712, -12.0124) (-20.3098, -12.0395) (-20.3566, -12.0754) (-20.4025, -12.1128) (-20.4478, -12.1511) (-20.4928, -12.1899) (-20.5376, -12.2291) (-20.5821, -12.2686) (-20.6263, -12.3085) (-20.6701, -12.3491) (-20.7134, -12.3903) (-20.7562, -12.4323) (-20.7985, -12.4749) (-20.8405, -12.518) (-20.8821, -12.5616) (-20.9234, -12.6056) (-20.9644, -12.65) (-21.0051, -12.6947) (-21.0456, -12.7398) (-21.0857, -12.7854) (-21.1255, -12.8313) (-21.1649, -12.8777) (-21.2041, -12.9245) (-21.2429, -12.9717) (-21.2815, -13.0192) (-21.3198, -13.0671) (-21.3577, -13.1152) (-21.3955, -13.1638) (-21.4329, -13.2126) (-21.4701, -13.2618) (-21.507, -13.3113) (-21.5436, -13.3612) (-21.5799, -13.4113) (-21.616, -13.4618) (-21.6518, -13.5126) (-21.6874, -13.5636) (-21.7227, -13.615) (-21.7577, -13.6666) (-21.7925, -13.7185) (-21.827, -13.7708) (-21.8612, -13.8233) (-21.8952, -13.876) (-21.929, -13.9291) (-21.9625, -13.9824) (-21.9957, -14.0359) (-22.0287, -14.0898) (-22.0615, -14.1439) (-22.0939, -14.1982) (-22.1262, -14.2528) (-22.1582, -14.3077) (-22.1899, -14.3628) (-22.2215, -14.4181) (-22.2527, -14.4737) (-22.2837, -14.5295) (-22.3145, -14.5856) (-22.345, -14.6419) (-22.3753, -14.6984) (-22.4054, -14.7552) (-22.4352, -14.8121) (-22.4648, -14.8694) (-22.4941, -14.9268) (-22.5232, -14.9844) (-22.5521, -15.0423) (-22.5807, -15.1004) (-22.6091, -15.1587) (-22.6372, -15.2172) (-22.6651, -15.276) (-22.6928, -15.3349) (-22.7147, -15.3822) (-22.7311, -15.4178) (-22.7419, -15.4415) (-22.7473, -15.4534) knots 0 0 0 0 0 0 0.01428571 0.02857143 0.04285714 0.05714286 0.07142857 0.08571429 0.1 0.11428571 0.12857143 0.14285714 0.15714286 0.17142857 0.18571429 0.2 0.21428571 0.22857143 0.24285714 0.25714286 0.27142857 0.28571429 0.3 0.31428571 0.32857143 0.34285714 0.35714286 0.37142857 0.38571429 0.4 0.41428571 0.42857143 0.44285714 0.45714286 0.47142857 0.48571429 0.5 0.51428571 0.52857143 0.54285714 0.55714286 0.57142857 0.58571429 0.6 0.61428571 0.62857143 0.64285714 0.65714286 0.67142857 0.68571429 0.7 0.71428571 0.72857143 0.74285714 0.75714286 0.77142857 0.78571429 0.8 0.81428571 0.82857143 0.84285714 0.85714286 0.87142857 0.88571429 0.9 0.91428571 0.92857143 0.94285714 0.95714286 0.97142857 0.98571429 1 1 1 1 1 1
  arc A10 (-22.7473, -15.4534) -> (-21.7264, -16.8586) centre (0, 0) ccw
  spline S5 degree 5 poles (-21.7264, -16.8586) (-21.7134, -16.8572) (-21.6875, -16.8542) (-21.6486, -16.8496) (-21.5968, -16.8434) (-21.5322, -16.8353) (-21.4677, -16.8269) (-21.4034, -16.8182) (-21.3392, -16.8092) (-21.2751, -16.7999) (-21.2111, -16.7904) (-21.1473, -16.7805) (-21.0836, -16.7704) (-21.02, -16.7599) (-20.9566, -16.7492) (-20.8934, -16.7382) (-20.8302, -16.7268) (-20.7673, -16.7152) (-20.7044, -16.7032) (-20.6418, -16.691) (-20.5792, -16.6784) (-20.5169, -16.6656) (-20.4547, -16.6524) (-20.3926, -16.6389) (-20.3307, -16.6251) (-20.269, -16.611) (-20.2074, -16.5966) (-20.146, -16.5818) (-20.0848, -16.5668) (-20.0238, -16.5514) (-19.9629, -16.5357) (-19.9022, -16.5197) (-19.8417, -16.5033) (-19.7814, -16.4866) (-19.7212, -16.4696) (-19.6613, -16.4522) (-19.6015, -16.4345) (-19.542, -16.4165) (-19.4826, -16.3981) (-19.4235, -16.3794) (-19.3646, -16.3604) (-19.3059, -16.3409) (-19.2474, -16.3211) (-19.1891, -16.301) (-19.1311, -16.2805) (-19.0732, -16.2596) (-19.0157, -16.2383) (-18.9583, -16.2167) (-18.9012, -16.1948) (-18.8444, -16.1724) (-18.7878, -16.1496) (-18.7315, -16.1264) (-18.6754, -16.1028) (-18.6197, -16.0787) (-18.5643, -16.0542) (-18.5092, -16.0293) (-18.4543, -16.004) (-18.3997, -15.9783) (-18.3454, -15.9522) (-18.2914, -15.9256) (-18.2378, -15.8985) (-18.1847, -15.8708) (-18.1321, -15.8424) (-18.08, -15.8132) (-18.0283, -15.7835) (-17.977, -15.7534) (-17.9259, -15.7229) (-17.8751, -15.6921) (-17.8247, -15.6609) (-17.775, -15.6288) (-17.7263, -15.5953) (-17.6886, -15.567) (-17.6611, -15.5447) (-17.6432, -15.5294) (-17.6343, -15.5216) knots -1 -1 -1 -1 -1 -1 -0.98571429 -0.97142857 -0.95714286 -0.94285714 -0.92857143 -0.91428571 -0.9 -0.88571429 -0.87142857 -0.85714286 -0.84285714 -0.82857143 -0.81428571 -0.8 -0.78571429 -0.77142857 -0.75714286 -0.74285714 -0.72857143 -0.71428571 -0.7 -0.68571429 -0.67142857 -0.65714286 -0.64285714 -0.62857143 -0.61428571 -0.6 -0.58571429 -0.57142857 -0.55714286 -0.54285714 -0.52857143 -0.51428571 -0.5 -0.48571429 -0.47142857 -0.45714286 -0.44285714 -0.42857143 -0.41428571 -0.4 -0.38571429 -0.37142857 -0.35714286 -0.34285714 -0.32857143 -0.31428571 -0.3 -0.28571429 -0.27142857 -0.25714286 -0.24285714 -0.22857143 -0.21428571 -0.2 -0.18571429 -0.17142857 -0.15714286 -0.14285714 -0.12857143 -0.11428571 -0.1 -0.08571429 -0.07142857 -0.05714286 -0.04285714 -0.02857143 -0.01428571 0 0 0 0 0 0
  line L5 (-17.6343, -15.5216) -> (-17.2096, -15.1482)
  arc A11 (-15.8282, -15.2064) -> (-17.2096, -15.1482) centre (-16.5493, -15.8992) ccw
  arc A12 (-15.8282, -15.2064) -> (-15.2064, -15.8282) centre (0, 0) ccw
  arc A13 (-15.1482, -17.2096) -> (-15.2064, -15.8282) centre (-15.8992, -16.5493) ccw
  line L6 (-15.1482, -17.2096) -> (-15.5216, -17.6343)
  spline S6 degree 5 poles (-15.5216, -17.6343) (-15.5294, -17.6432) (-15.5447, -17.6611) (-15.567, -17.6886) (-15.5953, -17.7263) (-15.6288, -17.775) (-15.6609, -17.8247) (-15.6921, -17.8751) (-15.7229, -17.9259) (-15.7534, -17.977) (-15.7835, -18.0283) (-15.8132, -18.08) (-15.8424, -18.1321) (-15.8708, -18.1847) (-15.8985, -18.2378) (-15.9256, -18.2914) (-15.9522, -18.3454) (-15.9783, -18.3997) (-16.004, -18.4543) (-16.0293, -18.5092) (-16.0542, -18.5643) (-16.0787, -18.6197) (-16.1028, -18.6754) (-16.1264, -18.7315) (-16.1496, -18.7878) (-16.1724, -18.8444) (-16.1948, -18.9012) (-16.2167, -18.9583) (-16.2383, -19.0157) (-16.2596, -19.0732) (-16.2805, -19.1311) (-16.301, -19.1891) (-16.3211, -19.2474) (-16.3409, -19.3059) (-16.3604, -19.3646) (-16.3794, -19.4235) (-16.3981, -19.4826) (-16.4165, -19.542) (-16.4345, -19.6015) (-16.4522, -19.6613) (-16.4696, -19.7212) (-16.4866, -19.7814) (-16.5033, -19.8417) (-16.5197, -19.9022) (-16.5357, -19.9629) (-16.5514, -20.0238) (-16.5668, -20.0848) (-16.5818, -20.146) (-16.5966, -20.2074) (-16.611, -20.269) (-16.6251, -20.3307) (-16.6389, -20.3926) (-16.6524, -20.4547) (-16.6656, -20.5169) (-16.6784, -20.5792) (-16.691, -20.6418) (-16.7032, -20.7044) (-16.7152, -20.7673) (-16.7268, -20.8302) (-16.7382, -20.8934) (-16.7492, -20.9566) (-16.7599, -21.02) (-16.7704, -21.0836) (-16.7805, -21.1473) (-16.7904, -21.2111) (-16.7999, -21.2751) (-16.8092, -21.3392) (-16.8182, -21.4034) (-16.8269, -21.4677) (-16.8353, -21.5322) (-16.8434, -21.5968) (-16.8496, -21.6486) (-16.8542, -21.6875) (-16.8572, -21.7134) (-16.8586, -21.7264) knots 0 0 0 0 0 0 0.01428571 0.02857143 0.04285714 0.05714286 0.07142857 0.08571429 0.1 0.11428571 0.12857143 0.14285714 0.15714286 0.17142857 0.18571429 0.2 0.21428571 0.22857143 0.24285714 0.25714286 0.27142857 0.28571429 0.3 0.31428571 0.32857143 0.34285714 0.35714286 0.37142857 0.38571429 0.4 0.41428571 0.42857143 0.44285714 0.45714286 0.47142857 0.48571429 0.5 0.51428571 0.52857143 0.54285714 0.55714286 0.57142857 0.58571429 0.6 0.61428571 0.62857143 0.64285714 0.65714286 0.67142857 0.68571429 0.7 0.71428571 0.72857143 0.74285714 0.75714286 0.77142857 0.78571429 0.8 0.81428571 0.82857143 0.84285714 0.85714286 0.87142857 0.88571429 0.9 0.91428571 0.92857143 0.94285714 0.95714286 0.97142857 0.98571429 1 1 1 1 1 1
  arc A14 (-16.8586, -21.7264) -> (-15.4534, -22.7473) centre (0, 0) ccw
  spline S7 degree 5 poles (-15.4534, -22.7473) (-15.4415, -22.7419) (-15.4178, -22.7311) (-15.3822, -22.7147) (-15.3349, -22.6928) (-15.276, -22.6651) (-15.2172, -22.6372) (-15.1587, -22.6091) (-15.1004, -22.5807) (-15.0423, -22.5521) (-14.9844, -22.5232) (-14.9268, -22.4941) (-14.8694, -22.4648) (-14.8121, -22.4352) (-14.7552, -22.4054) (-14.6984, -22.3753) (-14.6419, -22.345) (-14.5856, -22.3145) (-14.5295, -22.2837) (-14.4737, -22.2527) (-14.4181, -22.2215) (-14.3628, -22.1899) (-14.3077, -22.1582) (-14.2528, -22.1262) (-14.1982, -22.0939) (-14.1439, -22.0615) (-14.0898, -22.0287) (-14.0359, -21.9957) (-13.9824, -21.9625) (-13.9291, -21.929) (-13.876, -21.8952) (-13.8233, -21.8612) (-13.7708, -21.827) (-13.7185, -21.7925) (-13.6666, -21.7577) (-13.615, -21.7227) (-13.5636, -21.6874) (-13.5126, -21.6518) (-13.4618, -21.616) (-13.4113, -21.5799) (-13.3612, -21.5436) (-13.3113, -21.507) (-13.2618, -21.4701) (-13.2126, -21.4329) (-13.1638, -21.3955) (-13.1152, -21.3577) (-13.0671, -21.3198) (-13.0192, -21.2815) (-12.9717, -21.2429) (-12.9245, -21.2041) (-12.8777, -21.1649) (-12.8313, -21.1255) (-12.7854, -21.0857) (-12.7398, -21.0456) (-12.6947, -21.0051) (-12.65, -20.9644) (-12.6056, -20.9234) (-12.5616, -20.8821) (-12.518, -20.8405) (-12.4749, -20.7985) (-12.4323, -20.7562) (-12.3903, -20.7134) (-12.3491, -20.6701) (-12.3085, -20.6263) (-12.2686, -20.5821) (-12.2291, -20.5376) (-12.1899, -20.4928) (-12.1511, -20.4478) (-12.1128, -20.4025) (-12.0754, -20.3566) (-12.0395, -20.3098) (-12.0124, -20.2712) (-11.9931, -20.2415) (-11.9808, -20.2214) (-11.9748, -20.2112) knots -1 -1 -1 -1 -1 -1 -0.98571429 -0.97142857 -0.95714286 -0.94285714 -0.92857143 -0.91428571 -0.9 -0.88571429 -0.87142857 -0.85714286 -0.84285714 -0.82857143 -0.81428571 -0.8 -0.78571429 -0.77142857 -0.75714286 -0.74285714 -0.72857143 -0.71428571 -0.7 -0.68571429 -0.67142857 -0.65714286 -0.64285714 -0.62857143 -0.61428571 -0.6 -0.58571429 -0.57142857 -0.55714286 -0.54285714 -0.52857143 -0.51428571 -0.5 -0.48571429 -0.47142857 -0.45714286 -0.44285714 -0.42857143 -0.41428571 -0.4 -0.38571429 -0.37142857 -0.35714286 -0.34285714 -0.32857143 -0.31428571 -0.3 -0.28571429 -0.27142857 -0.25714286 -0.24285714 -0.22857143 -0.21428571 -0.2 -0.18571429 -0.17142857 -0.15714286 -0.14285714 -0.12857143 -0.11428571 -0.1 -0.08571429 -0.07142857 -0.05714286 -0.04285714 -0.02857143 -0.01428571 0 0 0 0 0 0
  line L7 (-11.9748, -20.2112) -> (-11.6862, -19.7248)
  arc A15 (-10.3545, -19.3534) -> (-11.6862, -19.7248) centre (-10.8262, -20.2351) ccw
  arc A16 (-10.3545, -19.3534) -> (-9.571, -19.7526) centre (0, 0) ccw
  arc A17 (-9.0887, -21.0483) -> (-9.571, -19.7526) centre (-10.007, -20.6525) ccw
  line L8 (-9.0887, -21.0483) -> (-9.3126, -21.5677)
  spline S8 degree 5 poles (-9.3126, -21.5677) (-9.3173, -21.5785) (-9.3263, -21.6003) (-9.339, -21.6333) (-9.3543, -21.6779) (-9.3711, -21.7346) (-9.3863, -21.7918) (-9.4004, -21.8494) (-9.414, -21.9072) (-9.4272, -21.9652) (-9.44, -22.0233) (-9.4523, -22.0817) (-9.4638, -22.1402) (-9.4746, -22.199) (-9.4846, -22.2581) (-9.4938, -22.3175) (-9.5024, -22.377) (-9.5104, -22.4367) (-9.518, -22.4966) (-9.5251, -22.5566) (-9.5318, -22.6167) (-9.5379, -22.677) (-9.5436, -22.7374) (-9.5488, -22.798) (-9.5535, -22.8587) (-9.5576, -22.9196) (-9.5613, -22.9806) (-9.5646, -23.0417) (-9.5674, -23.1029) (-9.5698, -23.1642) (-9.5718, -23.2257) (-9.5734, -23.2872) (-9.5746, -23.3488) (-9.5753, -23.4106) (-9.5756, -23.4724) (-9.5756, -23.5344) (-9.5751, -23.5964) (-9.5742, -23.6585) (-9.573, -23.7207) (-9.5713, -23.783) (-9.5693, -23.8454) (-9.5669, -23.9078) (-9.5642, -23.9704) (-9.561, -24.033) (-9.5575, -24.0956) (-9.5536, -24.1584) (-9.5494, -24.2212) (-9.5448, -24.2841) (-9.5398, -24.347) (-9.5345, -24.41) (-9.5289, -24.4731) (-9.5229, -24.5362) (-9.5165, -24.5994) (-9.5098, -24.6626) (-9.5028, -24.7259) (-9.4954, -24.7893) (-9.4877, -24.8527) (-9.4796, -24.9161) (-9.4712, -24.9796) (-9.4625, -25.0432) (-9.4535, -25.1067) (-9.4441, -25.1704) (-9.4344, -25.234) (-9.4244, -25.2977) (-9.414, -25.3615) (-9.4033, -25.4253) (-9.3924, -25.4891) (-9.381, -25.5529) (-9.3694, -25.6168) (-9.3575, -25.6807) (-9.3452, -25.7447) (-9.3352, -25.7958) (-9.3275, -25.8342) (-9.3223, -25.8598) (-9.3197, -25.8726) knots 0 0 0 0 0 0 0.01428571 0.02857143 0.04285714 0.05714286 0.07142857 0.08571429 0.1 0.11428571 0.12857143 0.14285714 0.15714286 0.17142857 0.18571429 0.2 0.21428571 0.22857143 0.24285714 0.25714286 0.27142857 0.28571429 0.3 0.31428571 0.32857143 0.34285714 0.35714286 0.37142857 0.38571429 0.4 0.41428571 0.42857143 0.44285714 0.45714286 0.47142857 0.48571429 0.5 0.51428571 0.52857143 0.54285714 0.55714286 0.57142857 0.58571429 0.6 0.61428571 0.62857143 0.64285714 0.65714286 0.67142857 0.68571429 0.7 0.71428571 0.72857143 0.74285714 0.75714286 0.77142857 0.78571429 0.8 0.81428571 0.82857143 0.84285714 0.85714286 0.87142857 0.88571429 0.9 0.91428571 0.92857143 0.94285714 0.95714286 0.97142857 0.98571429 1 1 1 1 1 1
  arc A18 (-9.3197, -25.8726) -> (-7.6678, -26.4094) centre (0, 0) ccw
  spline S9 degree 5 poles (-7.6678, -26.4094) (-7.6581, -26.4006) (-7.6389, -26.3829) (-7.6101, -26.3563) (-7.5719, -26.3208) (-7.5244, -26.2763) (-7.4772, -26.2316) (-7.4302, -26.1868) (-7.3835, -26.1418) (-7.3371, -26.0966) (-7.291, -26.0513) (-7.2452, -26.0058) (-7.1996, -25.9602) (-7.1543, -25.9144) (-7.1093, -25.8684) (-7.0646, -25.8223) (-7.0202, -25.776) (-6.9761, -25.7296) (-6.9323, -25.683) (-6.8888, -25.6362) (-6.8456, -25.5893) (-6.8027, -25.5422) (-6.7601, -25.495) (-6.7179, -25.4476) (-6.6759, -25.4001) (-6.6343, -25.3524) (-6.5929, -25.3045) (-6.5519, -25.2565) (-6.5112, -25.2083) (-6.4709, -25.16) (-6.4309, -25.1115) (-6.3912, -25.0629) (-6.3519, -25.0141) (-6.3129, -24.9651) (-6.2742, -24.916) (-6.2359, -24.8667) (-6.198, -24.8173) (-6.1604, -24.7677) (-6.1232, -24.718) (-6.0864, -24.6681) (-6.0499, -24.618) (-6.0138, -24.5678) (-5.9781, -24.5174) (-5.9428, -24.4668) (-5.9079, -24.4161) (-5.8734, -24.3653) (-5.8393, -24.3142) (-5.8056, -24.263) (-5.7724, -24.2117) (-5.7395, -24.1602) (-5.7071, -24.1085) (-5.6752, -24.0566) (-5.6438, -24.0046) (-5.6129, -23.9523) (-5.5824, -23.9) (-5.5525, -23.8474) (-5.523, -23.7947) (-5.4939, -23.7418) (-5.4653, -23.6888) (-5.4372, -23.6355) (-5.4098, -23.5821) (-5.3831, -23.5284) (-5.3573, -23.4745) (-5.3322, -23.4203) (-5.3079, -23.3659) (-5.2841, -23.3114) (-5.2607, -23.2567) (-5.2377, -23.2019) (-5.2153, -23.147) (-5.1939, -23.0918) (-5.1742, -23.0361) (-5.1603, -22.9911) (-5.1512, -22.9569) (-5.1457, -22.9339) (-5.1431, -22.9224) knots -1 -1 -1 -1 -1 -1 -0.98571429 -0.97142857 -0.95714286 -0.94285714 -0.92857143 -0.91428571 -0.9 -0.88571429 -0.87142857 -0.85714286 -0.84285714 -0.82857143 -0.81428571 -0.8 -0.78571429 -0.77142857 -0.75714286 -0.74285714 -0.72857143 -0.71428571 -0.7 -0.68571429 -0.67142857 -0.65714286 -0.64285714 -0.62857143 -0.61428571 -0.6 -0.58571429 -0.57142857 -0.55714286 -0.54285714 -0.52857143 -0.51428571 -0.5 -0.48571429 -0.47142857 -0.45714286 -0.44285714 -0.42857143 -0.41428571 -0.4 -0.38571429 -0.37142857 -0.35714286 -0.34285714 -0.32857143 -0.31428571 -0.3 -0.28571429 -0.27142857 -0.25714286 -0.24285714 -0.22857143 -0.21428571 -0.2 -0.18571429 -0.17142857 -0.15714286 -0.14285714 -0.12857143 -0.11428571 -0.1 -0.08571429 -0.07142857 -0.05714286 -0.04285714 -0.02857143 -0.01428571 0 0 0 0 0 0
  line L9 (-5.1431, -22.9224) -> (-5.019, -22.3707)
  arc A19 (-3.8672, -21.6058) -> (-5.019, -22.3707) centre (-4.0434, -22.5902) ccw
  arc A20 (-3.8672, -21.6058) -> (-2.9987, -21.7434) centre (0, 0) ccw
  arc A21 (-2.1396, -22.8267) -> (-2.9987, -21.7434) centre (-3.1353, -22.734) ccw
  line L10 (-2.1396, -22.8267) -> (-2.192, -23.3898)